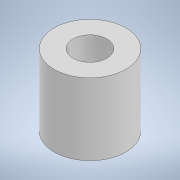
# Autodesk Inventor part: Bauteil1
Saved by Autodesk Inventor 2021 (Build 250183000, 183)
## iProperties
Created: 2021-06-03
Part Number: Bauteil1
Material: Generisch
Document SubType Name: Modeling
Designer: User
Density: 1 g/cm^3
Appearance: Vorgabe
Author: User
## iProperties of the stored document _3D-Druck.ipt
Created: 2021-06-03
Part Number: _3D-Druck
Material: Generisch
Document SubType Name: Modeling
Designer: User
Density: 1 g/cm^3
Appearance: Vorgabe
Author: User
Autodesk Inventor part; units mm, degrees
ref_plane "YZ Plane" through (0, 0, 0) normal (1, 0, 0) x (0, 1, 0)
ref_plane "XZ Plane" through (0, 0, 0) normal (0, 1, 0) x (-1, 0, 0)
ref_plane "XY Plane" through (0, 0, 0) normal (0, 0, 1) x (1, 0, 0)
sketch "Skizze1" plane through (0, 0, 0) normal (0, 0, 1) x (1, 0, 0)
  line L0 (0, -2.5) -> (0, 2.5)
  line L1 (-0.5, 0) -> (3, 0) projected
  line L2 (0, 2.5) -> (1.175, 2.5) construction
  line L3 (2.5, 2.5) -> (2.5, -2.5)
  line L4 (2.5, -2.5) -> (1.175, -2.5)
  line L5 (1.175, -2.5) -> (1.175, 2.5)
  line L6 (1.175, -2.5) -> (0, -2.5) construction
  line L7 (1.175, 2.5) -> (2.5, 2.5)
  point P0 (0, 0)
  dimension "d0" = 90
  dimension "d1" = 5
  dimension "d2" = 2.35
  dimension "d3" = 5
  constraints: 14 end point, 6 perpendicular, 1 midpoint
  measures "d0" angle of L0 L1
  measures "d1" diameter of L3 L0
  measures "d2" diameter of L5 L0
  measures "d3" distance between parallel lines of L2 L4
revolve "Umdrehung1" add sketch "Skizze1" angle 360 about axis through (0, -2.5, 0) along (0, 1, 0)
